Autodesk Inventor part; units mm, degrees
(part 2 of 3)
  spline S268 degree 2 poles (-6.9778, 47.9157) (-6.9778, 48.2091) (-7.3123, 48.8729) (-7.5541, 49.1508) knots 0 0 0 1 2 2 2
  line L188 (-7.5541, 49.1508) -> (-11.1151, 49.1508)
  line L189 (-11.1151, 49.1508) -> (-11.1151, 49.9535)
  line L190 (-11.1151, 49.9535) -> (-6.35, 49.9535)
  line L191 (-6.35, 54.8575) -> (-6.35, 54.0548)
  line L192 (-6.35, 54.0548) -> (-9.067, 54.0548)
  spline S269 degree 2 poles (-9.067, 54.0548) (-9.3964, 54.0548) (-9.9624, 53.993) (-10.1322, 53.9004) knots 0 0 0 1 2 2 2
  spline S270 degree 2 poles (-10.1322, 53.9004) (-10.3123, 53.8026) (-10.4873, 53.4527) (-10.4873, 53.1542) knots 0 0 0 1 2 2 2
  spline S271 degree 2 poles (-10.4873, 53.1542) (-10.4873, 52.8558) (-10.1682, 52.2228) (-9.9109, 51.9192) knots 0 0 0 1 2 2 2
  line L193 (-9.9109, 51.9192) -> (-6.35, 51.9192)
  line L194 (-6.35, 51.9192) -> (-6.35, 51.1165)
  line L195 (-6.35, 51.1165) -> (-11.1151, 51.1165)
  line L196 (-11.1151, 51.1165) -> (-11.1151, 51.9192)
  line L197 (-11.1151, 51.9192) -> (-10.585, 51.9192)
  spline S272 degree 2 poles (-10.585, 51.9192) (-10.9092, 52.2794) (-11.2489, 52.9741) (-11.2489, 53.3652) knots 0 0 0 1 2 2 2
  spline S273 degree 2 poles (-11.2489, 53.3652) (-11.2489, 54.0651) (-10.3226, 54.8575) (-9.4427, 54.8575) knots 0 0 0 1 2 2 2
  line L198 (-9.4427, 54.8575) -> (-6.35, 54.8575)
  spline S274 degree 2 poles (-6.2574, 57.4253) (-6.2574, 56.7718) (-7.0035, 56.0359) (-7.8114, 56.0359) knots 0 0 0 1 2 2 2
  line L199 (-7.8114, 56.0359) -> (-10.4513, 56.0359)
  line L200 (-10.4513, 56.0359) -> (-10.4513, 55.4956)
  line L201 (-10.4513, 55.4956) -> (-11.1151, 55.4956)
  line L202 (-11.1151, 55.4956) -> (-11.1151, 56.0359)
  line L203 (-11.1151, 56.0359) -> (-12.4839, 56.0359)
  line L204 (-12.4839, 56.0359) -> (-12.4839, 56.8387)
  line L205 (-12.4839, 56.8387) -> (-11.1151, 56.8387)
  line L206 (-11.1151, 56.8387) -> (-11.1151, 58.3155)
  line L207 (-11.1151, 58.3155) -> (-10.4513, 58.3155)
  line L208 (-10.4513, 58.3155) -> (-10.4513, 56.8387)
  line L209 (-10.4513, 56.8387) -> (-8.1819, 56.8387)
  spline S275 degree 2 poles (-8.1819, 56.8387) (-7.8217, 56.8387) (-7.4255, 56.8644) (-7.2557, 56.9519) knots 0 0 0 1 2 2 2
  spline S276 degree 2 poles (-7.2557, 56.9519) (-7.1064, 57.0239) (-6.9572, 57.3481) (-6.9572, 57.626) knots 0 0 0 1 2 2 2
  spline S277 degree 2 poles (-6.9572, 57.626) (-6.9572, 57.8215) (-7.0756, 58.1869) (-7.1116, 58.2692) knots 0 0 0 1 2 2 2
  line L210 (-7.1116, 58.2692) -> (-7.1116, 58.3155)
  line L211 (-7.1116, 58.3155) -> (-6.3912, 58.3155)
  spline S278 degree 2 poles (-6.3912, 58.3155) (-6.3294, 58.0891) (-6.2574, 57.626) (-6.2574, 57.4253) knots 0 0 0 1 2 2 2
  line L212 (-6.35, 63.5129) -> (-6.35, 62.566)
  line L213 (-6.35, 62.566) -> (-11.8252, 59.7564)
  line L214 (-11.8252, 59.7564) -> (-6.35, 59.7564)
  line L215 (-6.35, 59.7564) -> (-6.35, 58.9691)
  line L216 (-6.35, 58.9691) -> (-12.7, 58.9691)
  line L217 (-12.7, 58.9691) -> (-12.7, 60.1681)
  line L218 (-12.7, 60.1681) -> (-7.6725, 62.7255)
  line L219 (-7.6725, 62.7255) -> (-12.7, 62.7255)
  line L220 (-12.7, 62.7255) -> (-12.7, 63.5129)
  line L221 (-12.7, 63.5129) -> (-6.35, 63.5129)
  spline S279 degree 2 poles (-8.7325, 68.6536) (-7.5284, 68.6536) (-6.2162, 67.4958) (-6.2162, 66.5283) knots 0 0 0 1 2 2 2
  spline S280 degree 2 poles (-6.2162, 66.5283) (-6.2162, 65.5352) (-7.5696, 64.398) (-8.7325, 64.398) knots 0 0 0 1 2 2 2
  spline S281 degree 2 poles (-8.7325, 64.398) (-9.9264, 64.398) (-11.2489, 65.5712) (-11.2489, 66.5283) knots 0 0 0 1 2 2 2
  spline S282 degree 2 poles (-11.2489, 66.5283) (-11.2489, 67.4958) (-9.9315, 68.6536) (-8.7325, 68.6536) knots 0 0 0 1 2 2 2
  spline S283 degree 2 poles (-8.7325, 67.8251) (-9.6588, 67.8251) (-10.5593, 67.151) (-10.5593, 66.5283) knots 0 0 0 1 2 2 2
  spline S284 degree 2 poles (-10.5593, 66.5283) (-10.5593, 65.9057) (-9.6588, 65.2264) (-8.7325, 65.2264) knots 0 0 0 1 2 2 2
  spline S285 degree 2 poles (-8.7325, 65.2264) (-7.832, 65.2264) (-6.9058, 65.9057) (-6.9058, 66.5283) knots 0 0 0 1 2 2 2
  spline S286 degree 2 poles (-6.9058, 66.5283) (-6.9058, 67.1458) (-7.8166, 67.8251) (-8.7325, 67.8251) knots 0 0 0 1 2 2 2
  line L222 (-11.1151, 73.218) -> (-6.35, 71.4221)
  line L223 (-6.35, 71.4221) -> (-6.35, 70.7016)
  line L224 (-6.35, 70.7016) -> (-11.1151, 68.9212)
  line L225 (-11.1151, 68.9212) -> (-11.1151, 69.7908)
  line L226 (-11.1151, 69.7908) -> (-7.4461, 71.0927)
  line L227 (-7.4461, 71.0927) -> (-11.1151, 72.3843)
  line L228 (-11.1151, 72.3843) -> (-11.1151, 73.218)
  line L229 (-6.35, 77.6228) -> (-6.35, 73.7068)
  line L230 (-6.35, 73.7068) -> (-7.2505, 73.7068)
  spline S287 degree 2 poles (-7.2505, 73.7068) (-7.6468, 74.1288) (-8.3826, 74.8801) (-8.7788, 75.2403) knots 0 0 0 1 2 2 2
  spline S288 degree 2 poles (-8.7788, 75.2403) (-9.5765, 75.9659) (-10.5336, 76.4959) (-11.043, 76.4959) knots 0 0 0 1 2 2 2
  spline S289 degree 2 poles (-11.043, 76.4959) (-11.3106, 76.4959) (-11.712, 76.3312) (-11.8406, 76.182) knots 0 0 0 1 2 2 2
  spline S290 degree 2 poles (-11.8406, 76.182) (-11.9693, 76.0328) (-12.0979, 75.6417) (-12.0979, 75.405) knots 0 0 0 1 2 2 2
  spline S291 degree 2 poles (-12.0979, 75.405) (-12.0979, 75.1785) (-11.9847, 74.7154) (-11.8972, 74.5044) knots 0 0 0 1 2 2 2
  spline S292 degree 2 poles (-11.8972, 74.5044) (-11.8252, 74.3243) (-11.6194, 73.9899) (-11.5473, 73.8869) knots 0 0 0 1 2 2 2
  line L231 (-11.5473, 73.8869) -> (-11.5473, 73.8406)
  line L232 (-11.5473, 73.8406) -> (-12.453, 73.8406)
  spline S293 degree 2 poles (-12.453, 73.8406) (-12.5816, 74.1031) (-12.8338, 75.0448) (-12.8338, 75.4667) knots 0 0 0 1 2 2 2
  spline S294 degree 2 poles (-12.8338, 75.4667) (-12.8338, 76.3569) (-11.8921, 77.3604) (-11.0893, 77.3604) knots 0 0 0 1 2 2 2
  spline S295 degree 2 poles (-11.0893, 77.3604) (-10.7137, 77.3604) (-10.0859, 77.1854) (-9.8183, 77.0311) knots 0 0 0 1 2 2 2
  spline S296 degree 2 poles (-9.8183, 77.0311) (-9.5404, 76.8767) (-8.995, 76.429) (-8.7325, 76.182) knots 0 0 0 1 2 2 2
  spline S297 degree 2 poles (-8.7325, 76.182) (-8.2951, 75.7806) (-7.3586, 74.7978) (-7.0859, 74.5044) knots 0 0 0 1 2 2 2
  line L233 (-7.0859, 74.5044) -> (-7.0859, 77.6228)
  line L234 (-7.0859, 77.6228) -> (-6.35, 77.6228)
  spline S298 degree 2 poles (-9.525, 82.4239) (-7.8166, 82.4239) (-6.2162, 81.4308) (-6.2162, 80.3965) knots 0 0 0 1 2 2 2
  spline S299 degree 2 poles (-6.2162, 80.3965) (-6.2162, 79.3467) (-7.8474, 78.3638) (-9.5199, 78.3638) knots 0 0 0 1 2 2 2
  spline S300 degree 2 poles (-9.5199, 78.3638) (-11.2386, 78.3638) (-12.8286, 79.357) (-12.8286, 80.3965) knots 0 0 0 1 2 2 2
  spline S301 degree 2 poles (-12.8286, 80.3965) (-12.8286, 81.4411) (-11.182, 82.4239) (-9.525, 82.4239) knots 0 0 0 1 2 2 2
  spline S302 degree 2 poles (-7.5902, 81.333) (-7.9041, 81.4565) (-8.8715, 81.5594) (-9.525, 81.5594) knots 0 0 0 1 2 2 2
  spline S303 degree 2 poles (-9.525, 81.5594) (-10.1785, 81.5594) (-11.1408, 81.4565) (-11.465, 81.3279) knots 0 0 0 1 2 2 2
  spline S304 degree 2 poles (-11.465, 81.3279) (-11.7892, 81.1992) (-12.1237, 80.7515) (-12.1237, 80.3965) knots 0 0 0 1 2 2 2
  spline S305 degree 2 poles (-12.1237, 80.3965) (-12.1237, 80.0414) (-11.7892, 79.5834) (-11.4547, 79.4496) knots 0 0 0 1 2 2 2
  spline S306 degree 2 poles (-11.4547, 79.4496) (-11.1305, 79.321) (-10.1425, 79.2283) (-9.5199, 79.2283) knots 0 0 0 1 2 2 2
  spline S307 degree 2 poles (-9.5199, 79.2283) (-8.8509, 79.2283) (-7.9555, 79.3107) (-7.6056, 79.4445) knots 0 0 0 1 2 2 2
  spline S308 degree 2 poles (-7.6056, 79.4445) (-7.2763, 79.568) (-6.9212, 80.026) (-6.9212, 80.3965) knots 0 0 0 1 2 2 2
  spline S309 degree 2 poles (-6.9212, 80.3965) (-6.9212, 80.7464) (-7.2557, 81.2044) (-7.5902, 81.333) knots 0 0 0 1 2 2 2
  line L235 (-6.35, 87.153) -> (-6.35, 83.237)
  line L236 (-6.35, 83.237) -> (-7.2505, 83.237)
  spline S310 degree 2 poles (-7.2505, 83.237) (-7.6468, 83.6589) (-8.3826, 84.4102) (-8.7788, 84.7704) knots 0 0 0 1 2 2 2
  spline S311 degree 2 poles (-8.7788, 84.7704) (-9.5765, 85.496) (-10.5336, 86.026) (-11.043, 86.026) knots 0 0 0 1 2 2 2
  spline S312 degree 2 poles (-11.043, 86.026) (-11.3106, 86.026) (-11.712, 85.8614) (-11.8406, 85.7121) knots 0 0 0 1 2 2 2
  spline S313 degree 2 poles (-11.8406, 85.7121) (-11.9693, 85.5629) (-12.0979, 85.1718) (-12.0979, 84.9351) knots 0 0 0 1 2 2 2
  spline S314 degree 2 poles (-12.0979, 84.9351) (-12.0979, 84.7087) (-11.9847, 84.2456) (-11.8972, 84.0346) knots 0 0 0 1 2 2 2
  spline S315 degree 2 poles (-11.8972, 84.0346) (-11.8252, 83.8545) (-11.6194, 83.52) (-11.5473, 83.4171) knots 0 0 0 1 2 2 2
  line L237 (-11.5473, 83.4171) -> (-11.5473, 83.3708)
  line L238 (-11.5473, 83.3708) -> (-12.453, 83.3708)
  spline S316 degree 2 poles (-12.453, 83.3708) (-12.5816, 83.6332) (-12.8338, 84.5749) (-12.8338, 84.9969) knots 0 0 0 1 2 2 2
  spline S317 degree 2 poles (-12.8338, 84.9969) (-12.8338, 85.8871) (-11.8921, 86.8905) (-11.0893, 86.8905) knots 0 0 0 1 2 2 2
  spline S318 degree 2 poles (-11.0893, 86.8905) (-10.7137, 86.8905) (-10.0859, 86.7156) (-9.8183, 86.5612) knots 0 0 0 1 2 2 2
  spline S319 degree 2 poles (-9.8183, 86.5612) (-9.5404, 86.4068) (-8.995, 85.9591) (-8.7325, 85.7121) knots 0 0 0 1 2 2 2
  spline S320 degree 2 poles (-8.7325, 85.7121) (-8.2951, 85.3108) (-7.3586, 84.3279) (-7.0859, 84.0346) knots 0 0 0 1 2 2 2
  line L239 (-7.0859, 84.0346) -> (-7.0859, 87.153)
  line L240 (-7.0859, 87.153) -> (-6.35, 87.153)
  spline S321 degree 2 poles (-9.525, 91.9541) (-7.8166, 91.9541) (-6.2162, 90.9609) (-6.2162, 89.9266) knots 0 0 0 1 2 2 2
  spline S322 degree 2 poles (-6.2162, 89.9266) (-6.2162, 88.8768) (-7.8474, 87.894) (-9.5199, 87.894) knots 0 0 0 1 2 2 2
  spline S323 degree 2 poles (-9.5199, 87.894) (-11.2386, 87.894) (-12.8286, 88.8871) (-12.8286, 89.9266) knots 0 0 0 1 2 2 2
  spline S324 degree 2 poles (-12.8286, 89.9266) (-12.8286, 90.9712) (-11.182, 91.9541) (-9.525, 91.9541) knots 0 0 0 1 2 2 2
  spline S325 degree 2 poles (-7.5902, 90.8631) (-7.9041, 90.9866) (-8.8715, 91.0896) (-9.525, 91.0896) knots 0 0 0 1 2 2 2
  spline S326 degree 2 poles (-9.525, 91.0896) (-10.1785, 91.0896) (-11.1408, 90.9866) (-11.465, 90.858) knots 0 0 0 1 2 2 2
  spline S327 degree 2 poles (-11.465, 90.858) (-11.7892, 90.7294) (-12.1237, 90.2817) (-12.1237, 89.9266) knots 0 0 0 1 2 2 2
  spline S328 degree 2 poles (-12.1237, 89.9266) (-12.1237, 89.5715) (-11.7892, 89.1136) (-11.4547, 88.9798) knots 0 0 0 1 2 2 2
  spline S329 degree 2 poles (-11.4547, 88.9798) (-11.1305, 88.8511) (-10.1425, 88.7585) (-9.5199, 88.7585) knots 0 0 0 1 2 2 2
  spline S330 degree 2 poles (-9.5199, 88.7585) (-8.8509, 88.7585) (-7.9555, 88.8408) (-7.6056, 88.9746) knots 0 0 0 1 2 2 2
  spline S331 degree 2 poles (-7.6056, 88.9746) (-7.2763, 89.0981) (-6.9212, 89.5561) (-6.9212, 89.9266) knots 0 0 0 1 2 2 2
  spline S332 degree 2 poles (-6.9212, 89.9266) (-6.9212, 90.2765) (-7.2557, 90.7345) (-7.5902, 90.8631) knots 0 0 0 1 2 2 2
  line L241 (-1.5346, -65.6741) -> (-1.5346, -65.7153)
  spline S333 degree 2 poles (-1.5346, -65.7153) (-1.5758, -65.8234) (-1.6478, -66.2247) (-1.6478, -66.3843) knots 0 0 0 1 2 2 2
  spline S334 degree 2 poles (-1.6478, -66.3843) (-1.6478, -66.8885) (-1.195, -67.3208) (-0.5981, -67.3208) knots 0 0 0 1 2 2 2
  line L242 (-0.5981, -67.3208) -> (-0.4385, -67.3208)
  line L243 (-0.4385, -67.3208) -> (-0.4385, -65.9932)
  line L244 (-0.4385, -65.9932) -> (0.2253, -65.9932)
  line L245 (0.2253, -65.9932) -> (0.2253, -67.2951)
  line L246 (0.2253, -67.2951) -> (4.3265, -67.2951)
  line L247 (4.3265, -67.2951) -> (4.3265, -68.0978)
  line L248 (4.3265, -68.0978) -> (0.2253, -68.0978)
  line L249 (0.2253, -68.0978) -> (0.2253, -68.6381)
  line L250 (0.2253, -68.6381) -> (-0.4385, -68.6381)
  line L251 (-0.4385, -68.6381) -> (-0.4385, -68.0978)
  line L252 (-0.4385, -68.0978) -> (-0.5981, -68.0978)
  spline S335 degree 2 poles (-0.5981, -68.0978) (-1.4523, -68.0978) (-2.3477, -67.2693) (-2.3477, -66.4975) knots 0 0 0 1 2 2 2
  spline S336 degree 2 poles (-2.3477, -66.4975) (-2.3477, -66.2762) (-2.3013, -65.8491) (-2.2705, -65.6741) knots 0 0 0 1 2 2 2
  line L253 (-2.2705, -65.6741) -> (-1.5346, -65.6741)
  line L254 (4.3265, -64.3979) -> (4.3265, -65.2007)
  line L255 (4.3265, -65.2007) -> (-0.4385, -65.2007)
  line L256 (-0.4385, -65.2007) -> (-0.4385, -64.3979)
  line L257 (-0.4385, -64.3979) -> (4.3265, -64.3979)
  line L258 (-1.231, -64.3413) -> (-1.231, -65.2522)
  line L259 (-1.231, -65.2522) -> (-2.0646, -65.2522)
  line L260 (-2.0646, -65.2522) -> (-2.0646, -64.3413)
  line L261 (-2.0646, -64.3413) -> (-1.231, -64.3413)
  line L262 (4.3265, -62.4014) -> (4.3265, -63.2041)
  line L263 (4.3265, -63.2041) -> (-2.3065, -63.2041)
  line L264 (-2.3065, -63.2041) -> (-2.3065, -62.4014)
  line L265 (-2.3065, -62.4014) -> (4.3265, -62.4014)
  spline S337 degree 2 poles (4.4346, -59.1543) (4.4346, -60.2967) (3.1533, -61.5523) (1.9697, -61.5523) knots 0 0 0 1 2 2 2
  spline S338 degree 2 poles (1.9697, -61.5523) (0.8068, -61.5523) (-0.5723, -60.3327) (-0.5723, -59.3499) knots 0 0 0 1 2 2 2
  spline S339 degree 2 poles (-0.5723, -59.3499) (-0.5723, -58.9073) (-0.315, -58.2229) (-0.0423, -57.9708) knots 0 0 0 1 2 2 2
  spline S340 degree 2 poles (-0.0423, -57.9708) (0.2304, -57.7135) (1.0177, -57.4407) (1.5889, -57.4407) knots 0 0 0 1 2 2 2
  line L266 (1.5889, -57.4407) -> (2.0263, -57.4407)
  line L267 (2.0263, -57.4407) -> (2.0263, -60.7392)
  spline S341 degree 2 poles (2.0263, -60.7392) (2.8548, -60.7392) (3.7348, -59.9056) (3.7348, -59.1646) knots 0 0 0 1 2 2 2
  spline S342 degree 2 poles (3.7348, -59.1646) (3.7348, -58.9022) (3.6164, -58.3927) (3.5238, -58.1869) knots 0 0 0 1 2 2 2
  spline S343 degree 2 poles (3.5238, -58.1869) (3.4209, -57.9708) (3.2408, -57.6723) (3.1584, -57.5745) knots 0 0 0 1 2 2 2
  line L268 (3.1584, -57.5745) -> (3.1584, -57.5282)
  line L269 (3.1584, -57.5282) -> (4.0332, -57.5282)
  spline S344 degree 2 poles (4.0332, -57.5282) (4.0898, -57.6672) (4.2545, -58.0891) (4.3008, -58.2538) knots 0 0 0 1 2 2 2
  spline S345 degree 2 poles (4.3008, -58.2538) (4.3677, -58.4853) (4.4346, -58.8661) (4.4346, -59.1543) knots 0 0 0 1 2 2 2
  spline S346 degree 2 poles (1.414, -58.2229) (1.0898, -58.2332) (0.6164, -58.367) (0.4568, -58.4956) knots 0 0 0 1 2 2 2
  spline S347 degree 2 poles (0.4568, -58.4956) (0.2767, -58.6346) (0.0863, -59.072) (0.0863, -59.3962) knots 0 0 0 1 2 2 2
  spline S348 degree 2 poles (0.0863, -59.3962) (0.0863, -59.7152) (0.2767, -60.1629) (0.462, -60.3482) knots 0 0 0 1 2 2 2
  spline S349 degree 2 poles (0.462, -60.3482) (0.6524, -60.5283) (1.1104, -60.7135) (1.414, -60.7392) knots 0 0 0 1 2 2 2
  line L270 (1.414, -60.7392) -> (1.414, -58.2229)
  line L271 (4.3265, -55.156) -> (4.3265, -56.1749)
  line L272 (4.3265, -56.1749) -> (3.1121, -56.1749)
  line L273 (3.1121, -56.1749) -> (3.1121, -55.156)
  line L274 (3.1121, -55.156) -> (4.3265, -55.156)
  line L275 (0.7759, -55.156) -> (0.7759, -56.1749)
  line L276 (0.7759, -56.1749) -> (-0.4385, -56.1749)
  line L277 (-0.4385, -56.1749) -> (-0.4385, -55.156)
  line L278 (-0.4385, -55.156) -> (0.7759, -55.156)
  spline S350 degree 2 poles (4.4346, -48.9192) (4.4346, -49.4132) (4.131, -50.2314) (3.8222, -50.5247) knots 0 0 0 1 2 2 2
  spline S351 degree 2 poles (3.8222, -50.5247) (3.5186, -50.818) (2.5821, -51.1422) (1.9543, -51.1422) knots 0 0 0 1 2 2 2
  spline S352 degree 2 poles (1.9543, -51.1422) (1.3265, -51.1422) (0.4105, -50.8077) (0.1018, -50.5247) knots 0 0 0 1 2 2 2
  spline S353 degree 2 poles (0.1018, -50.5247) (-0.2121, -50.2417) (-0.5466, -49.4029) (-0.5466, -48.9192) knots 0 0 0 1 2 2 2
  spline S354 degree 2 poles (-0.5466, -48.9192) (-0.5466, -48.5281) (-0.3253, -47.7974) (-0.1813, -47.5144) knots 0 0 0 1 2 2 2
  line L279 (-0.1813, -47.5144) -> (0.7193, -47.5144)
  line L280 (0.7193, -47.5144) -> (0.7193, -47.5607)
  spline S355 degree 2 poles (0.7193, -47.5607) (0.6472, -47.6482) (0.462, -47.9157) (0.3642, -48.1061) knots 0 0 0 1 2 2 2
  spline S356 degree 2 poles (0.3642, -48.1061) (0.2819, -48.2759) (0.1532, -48.7288) (0.1532, -48.9346) knots 0 0 0 1 2 2 2
  spline S357 degree 2 poles (0.1532, -48.9346) (0.1532, -49.5573) (1.0949, -50.3137) (1.9543, -50.3137) knots 0 0 0 1 2 2 2
  spline S358 degree 2 poles (1.9543, -50.3137) (2.7931, -50.3137) (3.7348, -49.583) (3.7348, -48.9346) knots 0 0 0 1 2 2 2
  spline S359 degree 2 poles (3.7348, -48.9346) (3.7348, -48.5435) (3.4106, -47.8334) (3.1584, -47.5607) knots 0 0 0 1 2 2 2
  line L281 (3.1584, -47.5607) -> (3.1584, -47.5144)
  line L282 (3.1584, -47.5144) -> (4.0589, -47.5144)
  spline S360 degree 2 poles (4.0589, -47.5144) (4.1155, -47.6327) (4.2751, -47.9929) (4.3111, -48.137) knots 0 0 0 1 2 2 2
  spline S361 degree 2 poles (4.3111, -48.137) (4.3728, -48.3428) (4.4346, -48.667) (4.4346, -48.9192) knots 0 0 0 1 2 2 2
  spline S362 degree 2 poles (1.944, -42.8676) (3.1481, -42.8676) (4.4603, -44.0255) (4.4603, -44.9929) knots 0 0 0 1 2 2 2
  spline S363 degree 2 poles (4.4603, -44.9929) (4.4603, -45.986) (3.107, -47.1233) (1.944, -47.1233) knots 0 0 0 1 2 2 2
  spline S364 degree 2 poles (1.944, -47.1233) (0.7502, -47.1233) (-0.5723, -45.95) (-0.5723, -44.9929) knots 0 0 0 1 2 2 2
  spline S365 degree 2 poles (-0.5723, -44.9929) (-0.5723, -44.0255) (0.745, -42.8676) (1.944, -42.8676) knots 0 0 0 1 2 2 2
  spline S366 degree 2 poles (1.944, -43.6961) (1.0177, -43.6961) (0.1172, -44.3702) (0.1172, -44.9929) knots 0 0 0 1 2 2 2
  spline S367 degree 2 poles (0.1172, -44.9929) (0.1172, -45.6155) (1.0177, -46.2948) (1.944, -46.2948) knots 0 0 0 1 2 2 2
  spline S368 degree 2 poles (1.944, -46.2948) (2.8445, -46.2948) (3.7708, -45.6155) (3.7708, -44.9929) knots 0 0 0 1 2 2 2
  spline S369 degree 2 poles (3.7708, -44.9929) (3.7708, -44.3754) (2.86, -43.6961) (1.944, -43.6961) knots 0 0 0 1 2 2 2
  line L283 (4.3265, -38.3033) -> (4.3265, -39.106)
  line L284 (4.3265, -39.106) -> (1.6095, -39.106)
  spline S370 degree 2 poles (1.6095, -39.106) (1.2802, -39.106) (0.7141, -39.1678) (0.5443, -39.2604) knots 0 0 0 1 2 2 2
  spline S371 degree 2 poles (0.5443, -39.2604) (0.3642, -39.3582) (0.1893, -39.7081) (0.1893, -40.0065) knots 0 0 0 1 2 2 2
  spline S372 degree 2 poles (0.1893, -40.0065) (0.1893, -40.305) (0.5083, -40.9379) (0.7656, -41.2415) knots 0 0 0 1 2 2 2
  line L285 (0.7656, -41.2415) -> (4.3265, -41.2415)
  line L286 (4.3265, -41.2415) -> (4.3265, -42.0443)
  line L287 (4.3265, -42.0443) -> (-0.4385, -42.0443)
  line L288 (-0.4385, -42.0443) -> (-0.4385, -41.2415)
  line L289 (-0.4385, -41.2415) -> (0.0915, -41.2415)
  spline S373 degree 2 poles (0.0915, -41.2415) (-0.2327, -40.8813) (-0.5723, -40.1866) (-0.5723, -39.7956) knots 0 0 0 1 2 2 2
  spline S374 degree 2 poles (-0.5723, -39.7956) (-0.5723, -39.0957) (0.3539, -38.3033) (1.2339, -38.3033) knots 0 0 0 1 2 2 2
  line L290 (1.2339, -38.3033) -> (4.3265, -38.3033)
  line L291 (4.3265, -33.4353) -> (4.3265, -34.238)
  line L292 (4.3265, -34.238) -> (1.6095, -34.238)
  spline S375 degree 2 poles (1.6095, -34.238) (1.2802, -34.238) (0.7141, -34.2998) (0.5443, -34.3924) knots 0 0 0 1 2 2 2
  spline S376 degree 2 poles (0.5443, -34.3924) (0.3642, -34.4902) (0.1893, -34.8401) (0.1893, -35.1386) knots 0 0 0 1 2 2 2
  spline S377 degree 2 poles (0.1893, -35.1386) (0.1893, -35.437) (0.5083, -36.07) (0.7656, -36.3736) knots 0 0 0 1 2 2 2
  line L293 (0.7656, -36.3736) -> (4.3265, -36.3736)
  line L294 (4.3265, -36.3736) -> (4.3265, -37.1763)
  line L295 (4.3265, -37.1763) -> (-0.4385, -37.1763)
  line L296 (-0.4385, -37.1763) -> (-0.4385, -36.3736)
  line L297 (-0.4385, -36.3736) -> (0.0915, -36.3736)
  spline S378 degree 2 poles (0.0915, -36.3736) (-0.2327, -36.0133) (-0.5723, -35.3187) (-0.5723, -34.9276) knots 0 0 0 1 2 2 2
  spline S379 degree 2 poles (-0.5723, -34.9276) (-0.5723, -34.2277) (0.3539, -33.4353) (1.2339, -33.4353) knots 0 0 0 1 2 2 2
  line L298 (1.2339, -33.4353) -> (4.3265, -33.4353)
  spline S380 degree 2 poles (4.4346, -30.2397) (4.4346, -31.3821) (3.1533, -32.6377) (1.9697, -32.6377) knots 0 0 0 1 2 2 2
  spline S381 degree 2 poles (1.9697, -32.6377) (0.8068, -32.6377) (-0.5723, -31.4181) (-0.5723, -30.4352) knots 0 0 0 1 2 2 2
  spline S382 degree 2 poles (-0.5723, -30.4352) (-0.5723, -29.9927) (-0.315, -29.3083) (-0.0423, -29.0561) knots 0 0 0 1 2 2 2
  spline S383 degree 2 poles (-0.0423, -29.0561) (0.2304, -28.7988) (1.0177, -28.5261) (1.5889, -28.5261) knots 0 0 0 1 2 2 2
  line L299 (1.5889, -28.5261) -> (2.0263, -28.5261)
  line L300 (2.0263, -28.5261) -> (2.0263, -31.8246)
  spline S384 degree 2 poles (2.0263, -31.8246) (2.8548, -31.8246) (3.7348, -30.991) (3.7348, -30.25) knots 0 0 0 1 2 2 2
  spline S385 degree 2 poles (3.7348, -30.25) (3.7348, -29.9875) (3.6164, -29.4781) (3.5238, -29.2723) knots 0 0 0 1 2 2 2
  spline S386 degree 2 poles (3.5238, -29.2723) (3.4209, -29.0561) (3.2408, -28.7577) (3.1584, -28.6599) knots 0 0 0 1 2 2 2
  line L301 (3.1584, -28.6599) -> (3.1584, -28.6136)
  line L302 (3.1584, -28.6136) -> (4.0332, -28.6136)
  spline S387 degree 2 poles (4.0332, -28.6136) (4.0898, -28.7525) (4.2545, -29.1745) (4.3008, -29.3392) knots 0 0 0 1 2 2 2
  spline S388 degree 2 poles (4.3008, -29.3392) (4.3677, -29.5707) (4.4346, -29.9515) (4.4346, -30.2397) knots 0 0 0 1 2 2 2
  spline S389 degree 2 poles (1.414, -29.3083) (1.0898, -29.3186) (0.6164, -29.4524) (0.4568, -29.581) knots 0 0 0 1 2 2 2
  spline S390 degree 2 poles (0.4568, -29.581) (0.2767, -29.72) (0.0863, -30.1574) (0.0863, -30.4815) knots 0 0 0 1 2 2 2
  spline S391 degree 2 poles (0.0863, -30.4815) (0.0863, -30.8006) (0.2767, -31.2483) (0.462, -31.4335) knots 0 0 0 1 2 2 2
  spline S392 degree 2 poles (0.462, -31.4335) (0.6524, -31.6136) (1.1104, -31.7989) (1.414, -31.8246) knots 0 0 0 1 2 2 2
  line L303 (1.414, -31.8246) -> (1.414, -29.3083)
  spline S393 degree 2 poles (4.4346, -25.8194) (4.4346, -26.3134) (4.131, -27.1316) (3.8222, -27.4249) knots 0 0 0 1 2 2 2
  spline S394 degree 2 poles (3.8222, -27.4249) (3.5186, -27.7182) (2.5821, -28.0424) (1.9543, -28.0424) knots 0 0 0 1 2 2 2
  spline S395 degree 2 poles (1.9543, -28.0424) (1.3265, -28.0424) (0.4105, -27.7079) (0.1018, -27.4249) knots 0 0 0 1 2 2 2
  spline S396 degree 2 poles (0.1018, -27.4249) (-0.2121, -27.1419) (-0.5466, -26.3031) (-0.5466, -25.8194) knots 0 0 0 1 2 2 2
  spline S397 degree 2 poles (-0.5466, -25.8194) (-0.5466, -25.4283) (-0.3253, -24.6976) (-0.1813, -24.4146) knots 0 0 0 1 2 2 2
  line L304 (-0.1813, -24.4146) -> (0.7193, -24.4146)
  line L305 (0.7193, -24.4146) -> (0.7193, -24.4609)
  spline S398 degree 2 poles (0.7193, -24.4609) (0.6472, -24.5484) (0.462, -24.8159) (0.3642, -25.0063) knots 0 0 0 1 2 2 2
  spline S399 degree 2 poles (0.3642, -25.0063) (0.2819, -25.1762) (0.1532, -25.629) (0.1532, -25.8348) knots 0 0 0 1 2 2 2
  spline S400 degree 2 poles (0.1532, -25.8348) (0.1532, -26.4575) (1.0949, -27.2139) (1.9543, -27.2139) knots 0 0 0 1 2 2 2
  spline S401 degree 2 poles (1.9543, -27.2139) (2.7931, -27.2139) (3.7348, -26.4832) (3.7348, -25.8348) knots 0 0 0 1 2 2 2
  spline S402 degree 2 poles (3.7348, -25.8348) (3.7348, -25.4437) (3.4106, -24.7336) (3.1584, -24.4609) knots 0 0 0 1 2 2 2
  line L306 (3.1584, -24.4609) -> (3.1584, -24.4146)
  line L307 (3.1584, -24.4146) -> (4.0589, -24.4146)
  spline S403 degree 2 poles (4.0589, -24.4146) (4.1155, -24.5329) (4.2751, -24.8931) (4.3111, -25.0372) knots 0 0 0 1 2 2 2
  spline S404 degree 2 poles (4.3111, -25.0372) (4.3728, -25.243) (4.4346, -25.5672) (4.4346, -25.8194) knots 0 0 0 1 2 2 2
  spline S405 degree 2 poles (4.4192, -22.243) (4.4192, -22.8965) (3.673, -23.6324) (2.8651, -23.6324) knots 0 0 0 1 2 2 2
  line L308 (2.8651, -23.6324) -> (0.2253, -23.6324)
  line L309 (0.2253, -23.6324) -> (0.2253, -24.1727)
  line L310 (0.2253, -24.1727) -> (-0.4385, -24.1727)
  line L311 (-0.4385, -24.1727) -> (-0.4385, -23.6324)
  line L312 (-0.4385, -23.6324) -> (-1.8073, -23.6324)
  line L313 (-1.8073, -23.6324) -> (-1.8073, -22.8296)
  line L314 (-1.8073, -22.8296) -> (-0.4385, -22.8296)
  line L315 (-0.4385, -22.8296) -> (-0.4385, -21.3528)
  line L316 (-0.4385, -21.3528) -> (0.2253, -21.3528)
  line L317 (0.2253, -21.3528) -> (0.2253, -22.8296)
  line L318 (0.2253, -22.8296) -> (2.4946, -22.8296)
  spline S406 degree 2 poles (2.4946, -22.8296) (2.8548, -22.8296) (3.251, -22.8039) (3.4209, -22.7164) knots 0 0 0 1 2 2 2
  spline S407 degree 2 poles (3.4209, -22.7164) (3.5701, -22.6444) (3.7193, -22.3202) (3.7193, -22.0423) knots 0 0 0 1 2 2 2
  spline S408 degree 2 poles (3.7193, -22.0423) (3.7193, -21.8468) (3.601, -21.4814) (3.5649, -21.3991) knots 0 0 0 1 2 2 2
  line L319 (3.5649, -21.3991) -> (3.5649, -21.3528)
  line L320 (3.5649, -21.3528) -> (4.2854, -21.3528)
  spline S409 degree 2 poles (4.2854, -21.3528) (4.3471, -21.5792) (4.4192, -22.0423) (4.4192, -22.243) knots 0 0 0 1 2 2 2
  spline S410 degree 2 poles (1.944, -16.845) (3.1481, -16.845) (4.4603, -18.0028) (4.4603, -18.9702) knots 0 0 0 1 2 2 2
  spline S411 degree 2 poles (4.4603, -18.9702) (4.4603, -19.9634) (3.107, -21.1006) (1.944, -21.1006) knots 0 0 0 1 2 2 2
  spline S412 degree 2 poles (1.944, -21.1006) (0.7502, -21.1006) (-0.5723, -19.9274) (-0.5723, -18.9702) knots 0 0 0 1 2 2 2
  spline S413 degree 2 poles (-0.5723, -18.9702) (-0.5723, -18.0028) (0.745, -16.845) (1.944, -16.845) knots 0 0 0 1 2 2 2
  spline S414 degree 2 poles (1.944, -17.6735) (1.0177, -17.6735) (0.1172, -18.3476) (0.1172, -18.9702) knots 0 0 0 1 2 2 2
  spline S415 degree 2 poles (0.1172, -18.9702) (0.1172, -19.5929) (1.0177, -20.2721) (1.944, -20.2721) knots 0 0 0 1 2 2 2
  spline S416 degree 2 poles (1.944, -20.2721) (2.8445, -20.2721) (3.7708, -19.5929) (3.7708, -18.9702) knots 0 0 0 1 2 2 2
  spline S417 degree 2 poles (3.7708, -18.9702) (3.7708, -18.3527) (2.86, -17.6735) (1.944, -17.6735) knots 0 0 0 1 2 2 2
  line L321 (0.4208, -13.495) -> (0.4208, -13.5362)
  spline S418 degree 2 poles (0.4208, -13.5362) (0.3951, -13.6288) (0.3848, -13.8295) (0.3848, -13.9685) knots 0 0 0 1 2 2 2
  spline S419 degree 2 poles (0.3848, -13.9685) (0.3848, -14.2926) (0.6678, -14.9307) (0.9457, -15.2189) knots 0 0 0 1 2 2 2
  line L322 (0.9457, -15.2189) -> (4.3265, -15.2189)
  line L323 (4.3265, -15.2189) -> (4.3265, -16.0217)
  line L324 (4.3265, -16.0217) -> (-0.4385, -16.0217)
  line L325 (-0.4385, -16.0217) -> (-0.4385, -15.2189)
  line L326 (-0.4385, -15.2189) -> (0.2716, -15.2189)
  spline S420 degree 2 poles (0.2716, -15.2189) (-0.1195, -14.7815) (-0.4385, -14.128) (-0.4385, -13.8192) knots 0 0 0 1 2 2 2
  spline S421 degree 2 poles (-0.4385, -13.8192) (-0.4385, -13.6957) (-0.4283, -13.5722) (-0.4128, -13.495) knots 0 0 0 1 2 2 2
  line L327 (-0.4128, -13.495) -> (0.4208, -13.495)
  line L328 (4.3265, -11.3286) -> (-1.2722, -11.3286)
  line L329 (-1.2722, -11.3286) -> (-1.2722, -13.459)
  line L330 (-1.2722, -13.459) -> (-2.0235, -13.459)
  line L331 (-2.0235, -13.459) -> (-2.0235, -8.3543)
  line L332 (-2.0235, -8.3543) -> (-1.2722, -8.3543)
  line L333 (-1.2722, -8.3543) -> (-1.2722, -10.4847)
  line L334 (-1.2722, -10.4847) -> (4.3265, -10.4847)
  line L335 (4.3265, -10.4847) -> (4.3265, -11.3286)
  spline S422 degree 2 poles (1.944, -3.8517) (3.1481, -3.8517) (4.4603, -5.0095) (4.4603, -5.9769) knots 0 0 0 1 2 2 2
  spline S423 degree 2 poles (4.4603, -5.9769) (4.4603, -6.9701) (3.107, -8.1073) (1.944, -8.1073) knots 0 0 0 1 2 2 2
  spline S424 degree 2 poles (1.944, -8.1073) (0.7502, -8.1073) (-0.5723, -6.9341) (-0.5723, -5.9769) knots 0 0 0 1 2 2 2
  spline S425 degree 2 poles (-0.5723, -5.9769) (-0.5723, -5.0095) (0.745, -3.8517) (1.944, -3.8517) knots 0 0 0 1 2 2 2
  spline S426 degree 2 poles (1.944, -4.6802) (1.0177, -4.6802) (0.1172, -5.3543) (0.1172, -5.9769) knots 0 0 0 1 2 2 2
  spline S427 degree 2 poles (0.1172, -5.9769) (0.1172, -6.5996) (1.0177, -7.2788) (1.944, -7.2788) knots 0 0 0 1 2 2 2
  spline S428 degree 2 poles (1.944, -7.2788) (2.8445, -7.2788) (3.7708, -6.5996) (3.7708, -5.9769) knots 0 0 0 1 2 2 2
  spline S429 degree 2 poles (3.7708, -5.9769) (3.7708, -5.3594) (2.86, -4.6802) (1.944, -4.6802) knots 0 0 0 1 2 2 2
  line L336 (4.3265, -1.4846) -> (-1.2722, -1.4846)
  line L337 (-1.2722, -1.4846) -> (-1.2722, -3.615)
  line L338 (-1.2722, -3.615) -> (-2.0235, -3.615)
  line L339 (-2.0235, -3.615) -> (-2.0235, 1.4897)
  line L340 (-2.0235, 1.4897) -> (-1.2722, 1.4897)
  line L341 (-1.2722, 1.4897) -> (-1.2722, -0.6407)
  line L342 (-1.2722, -0.6407) -> (4.3265, -0.6407)
  line L343 (4.3265, -0.6407) -> (4.3265, -1.4846)
  line L344 (4.3265, 5.7814) -> (4.3265, 4.9786)
  line L345 (4.3265, 4.9786) -> (3.8016, 4.9786)
  spline S430 degree 2 poles (3.8016, 4.9786) (4.1258, 4.6081) (4.4603, 3.9443) (4.4603, 3.5326) knots 0 0 0 1 2 2 2
  spline S431 degree 2 poles (4.4603, 3.5326) (4.4603, 3.2239) (4.2545, 2.6733) (4.0332, 2.4726) knots 0 0 0 1 2 2 2
  spline S432 degree 2 poles (4.0332, 2.4726) (3.8119, 2.2668) (3.1378, 2.0403) (2.6541, 2.0403) knots 0 0 0 1 2 2 2
  line L346 (2.6541, 2.0403) -> (-0.4385, 2.0403)
  line L347 (-0.4385, 2.0403) -> (-0.4385, 2.8431)
  line L348 (-0.4385, 2.8431) -> (2.2785, 2.8431)
  spline S433 degree 2 poles (2.2785, 2.8431) (2.6593, 2.8431) (3.1584, 2.8997) (3.3437, 2.9975) knots 0 0 0 1 2 2 2
  spline S434 degree 2 poles (3.3437, 2.9975) (3.5289, 3.0952) (3.6987, 3.4297) (3.6987, 3.7436) knots 0 0 0 1 2 2 2
  spline S435 degree 2 poles (3.6987, 3.7436) (3.6987, 4.0369) (3.3643, 4.7008) (3.1224, 4.9786) knots 0 0 0 1 2 2 2
  line L349 (3.1224, 4.9786) -> (-0.4385, 4.9786)
  line L350 (-0.4385, 4.9786) -> (-0.4385, 5.7814)
  line L351 (-0.4385, 5.7814) -> (4.3265, 5.7814)
  spline S436 degree 2 poles (1.8668, 10.9375) (3.0349, 10.9375) (4.4603, 9.8055) (4.4603, 8.9512) knots 0 0 0 1 2 2 2
  spline S437 degree 2 poles (4.4603, 8.9512) (4.4603, 8.5653) (4.2699, 8.0147) (4.1053, 7.7471) knots 0 0 0 1 2 2 2
  line L352 (4.1053, 7.7471) -> (4.3265, 7.6956)
  line L353 (4.3265, 7.6956) -> (4.3265, 6.9443)
  line L354 (4.3265, 6.9443) -> (-2.3065, 6.9443)
  line L355 (-2.3065, 6.9443) -> (-2.3065, 7.7471)
  line L356 (-2.3065, 7.7471) -> (0.0606, 7.7471)
  spline S438 degree 2 poles (0.0606, 7.7471) (-0.2121, 8.0507) (-0.5723, 8.7557) (-0.5723, 9.2034) knots 0 0 0 1 2 2 2
  spline S439 degree 2 poles (-0.5723, 9.2034) (-0.5723, 10.0113) (0.7193, 10.9375) (1.8668, 10.9375) knots 0 0 0 1 2 2 2
  spline S440 degree 2 poles (1.9286, 10.1091) (1.0743, 10.1091) (0.1893, 9.5893) (0.1893, 9.013) knots 0 0 0 1 2 2 2
  spline S441 degree 2 poles (0.1893, 9.013) (0.1893, 8.6888) (0.498, 8.0198) (0.7347, 7.7471) knots 0 0 0 1 2 2 2
  line L357 (0.7347, 7.7471) -> (3.4672, 7.7471)
  spline S442 degree 2 poles (3.4672, 7.7471) (3.6164, 8.0507) (3.7399, 8.519) (3.7399, 8.7969) knots 0 0 0 1 2 2 2
  spline S443 degree 2 poles (3.7399, 8.7969) (3.7399, 9.4092) (2.8702, 10.1091) (1.9286, 10.1091) knots 0 0 0 1 2 2 2
  spline S444 degree 2 poles (4.4346, 13.8398) (4.4346, 12.6974) (3.1533, 11.4418) (1.9697, 11.4418) knots 0 0 0 1 2 2 2
  spline S445 degree 2 poles (1.9697, 11.4418) (0.8068, 11.4418) (-0.5723, 12.6614) (-0.5723, 13.6443) knots 0 0 0 1 2 2 2
  spline S446 degree 2 poles (-0.5723, 13.6443) (-0.5723, 14.0868) (-0.315, 14.7712) (-0.0423, 15.0234) knots 0 0 0 1 2 2 2
  spline S447 degree 2 poles (-0.0423, 15.0234) (0.2304, 15.2807) (1.0177, 15.5534) (1.5889, 15.5534) knots 0 0 0 1 2 2 2
  line L358 (1.5889, 15.5534) -> (2.0263, 15.5534)
  line L359 (2.0263, 15.5534) -> (2.0263, 12.2549)
  spline S448 degree 2 poles (2.0263, 12.2549) (2.8548, 12.2549) (3.7348, 13.0885) (3.7348, 13.8295) knots 0 0 0 1 2 2 2
  spline S449 degree 2 poles (3.7348, 13.8295) (3.7348, 14.092) (3.6164, 14.6014) (3.5238, 14.8072) knots 0 0 0 1 2 2 2
  spline S450 degree 2 poles (3.5238, 14.8072) (3.4209, 15.0234) (3.2408, 15.3218) (3.1584, 15.4196) knots 0 0 0 1 2 2 2
  line L360 (3.1584, 15.4196) -> (3.1584, 15.4659)
  line L361 (3.1584, 15.4659) -> (4.0332, 15.4659)
  spline S451 degree 2 poles (4.0332, 15.4659) (4.0898, 15.327) (4.2545, 14.905) (4.3008, 14.7403) knots 0 0 0 1 2 2 2
  spline S452 degree 2 poles (4.3008, 14.7403) (4.3677, 14.5088) (4.4346, 14.128) (4.4346, 13.8398) knots 0 0 0 1 2 2 2
  spline S453 degree 2 poles (1.414, 14.7712) (1.0898, 14.7609) (0.6164, 14.6271) (0.4568, 14.4985) knots 0 0 0 1 2 2 2
  spline S454 degree 2 poles (0.4568, 14.4985) (0.2767, 14.3595) (0.0863, 13.9221) (0.0863, 13.598) knots 0 0 0 1 2 2 2
  spline S455 degree 2 poles (0.0863, 13.598) (0.0863, 13.2789) (0.2767, 12.8312) (0.462, 12.646) knots 0 0 0 1 2 2 2
  spline S456 degree 2 poles (0.462, 12.646) (0.6524, 12.4659) (1.1104, 12.2806) (1.414, 12.2549) knots 0 0 0 1 2 2 2
  line L362 (1.414, 12.2549) -> (1.414, 14.7712)
  spline S457 degree 2 poles (2.3762, 20.7353) (2.8497, 20.7353) (3.5752, 20.3751) (3.8119, 20.0766) knots 0 0 0 1 2 2 2
  spline S458 degree 2 poles (3.8119, 20.0766) (4.0898, 19.7164) (4.3265, 18.8982) (4.3265, 18.2498) knots 0 0 0 1 2 2 2
  line L363 (4.3265, 18.2498) -> (4.3265, 16.4282)
  line L364 (4.3265, 16.4282) -> (-2.0235, 16.4282)
  line L365 (-2.0235, 16.4282) -> (-2.0235, 18.1109)
  spline S459 degree 2 poles (-2.0235, 18.1109) (-2.0235, 18.7901) (-1.936, 19.4694) (-1.7662, 19.7781) knots 0 0 0 1 2 2 2
  spline S460 degree 2 poles (-1.7662, 19.7781) (-1.5861, 20.1229) (-0.9943, 20.4368) (-0.5929, 20.4368) knots 0 0 0 1 2 2 2
  spline S461 degree 2 poles (-0.5929, 20.4368) (-0.1452, 20.4368) (0.5649, 19.9634) (0.7656, 19.5466) knots 0 0 0 1 2 2 2
  line L366 (0.7656, 19.5466) -> (0.7965, 19.5466)
  spline S462 degree 2 poles (0.7965, 19.5466) (0.9508, 20.1126) (1.769, 20.7353) (2.3762, 20.7353) knots 0 0 0 1 2 2 2
  spline S463 degree 2 poles (2.4123, 19.8553) (2.0521, 19.8553) (1.5889, 19.6495) (1.4243, 19.3407) knots 0 0 0 1 2 2 2
  spline S464 degree 2 poles (1.4243, 19.3407) (1.3213, 19.1401) (1.2596, 18.6666) (1.2596, 18.2292) knots 0 0 0 1 2 2 2
  line L367 (1.2596, 18.2292) -> (1.2596, 17.2721)
  line L368 (1.2596, 17.2721) -> (3.6061, 17.2721)
  line L369 (3.6061, 17.2721) -> (3.6061, 17.9565)
  spline S465 degree 2 poles (3.6061, 17.9565) (3.6061, 18.5123) (3.5032, 19.1503) (3.3385, 19.3973) knots 0 0 0 1 2 2 2
  spline S466 degree 2 poles (3.3385, 19.3973) (3.1687, 19.6341) (2.7467, 19.8553) (2.4123, 19.8553) knots 0 0 0 1 2 2 2
  spline S467 degree 2 poles (-0.4746, 19.5569) (-0.701, 19.5569) (-1.0406, 19.4025) (-1.1384, 19.2327) knots 0 0 0 1 2 2 2
  spline S468 degree 2 poles (-1.1384, 19.2327) (-1.2516, 19.0268) (-1.3031, 18.5277) (-1.3031, 18.08) knots 0 0 0 1 2 2 2
  line L370 (-1.3031, 18.08) -> (-1.3031, 17.2721)
  line L371 (-1.3031, 17.2721) -> (0.5546, 17.2721)
  line L372 (0.5546, 17.2721) -> (0.5546, 18.2292)
  spline S469 degree 2 poles (0.5546, 18.2292) (0.5546, 18.6255) (0.4723, 19.0011) (0.3436, 19.2018) knots 0 0 0 1 2 2 2
  spline S470 degree 2 poles (0.3436, 19.2018) (0.2201, 19.3973) (-0.1761, 19.5569) (-0.4746, 19.5569) knots 0 0 0 1 2 2 2
  line L373 (0.4208, 24.0389) -> (0.4208, 23.9978)
  spline S471 degree 2 poles (0.4208, 23.9978) (0.3951, 23.9051) (0.3848, 23.7044) (0.3848, 23.5655) knots 0 0 0 1 2 2 2
  spline S472 degree 2 poles (0.3848, 23.5655) (0.3848, 23.2413) (0.6678, 22.6032) (0.9457, 22.3151) knots 0 0 0 1 2 2 2
  line L374 (0.9457, 22.3151) -> (4.3265, 22.3151)
  line L375 (4.3265, 22.3151) -> (4.3265, 21.5123)
  line L376 (4.3265, 21.5123) -> (-0.4385, 21.5123)
  line L377 (-0.4385, 21.5123) -> (-0.4385, 22.3151)
  line L378 (-0.4385, 22.3151) -> (0.2716, 22.3151)
  spline S473 degree 2 poles (0.2716, 22.3151) (-0.1195, 22.7525) (-0.4385, 23.406) (-0.4385, 23.7147) knots 0 0 0 1 2 2 2
  spline S474 degree 2 poles (-0.4385, 23.7147) (-0.4385, 23.8382) (-0.4283, 23.9617) (-0.4128, 24.0389) knots 0 0 0 1 2 2 2
  line L379 (-0.4128, 24.0389) -> (0.4208, 24.0389)
  spline S475 degree 2 poles (3.8222, 27.3168) (3.8943, 27.2191) (4.1516, 26.8897) (4.2288, 26.7354) knots 0 0 0 1 2 2 2
  spline S476 degree 2 poles (4.2288, 26.7354) (4.342, 26.5244) (4.4603, 26.1281) (4.4603, 25.7679) knots 0 0 0 1 2 2 2
  spline S477 degree 2 poles (4.4603, 25.7679) (4.4603, 25.4746) (4.239, 24.9446) (4.0384, 24.7439) knots 0 0 0 1 2 2 2
  spline S478 degree 2 poles (4.0384, 24.7439) (3.8428, 24.5535) (3.2665, 24.3219) (2.9474, 24.3219) knots 0 0 0 1 2 2 2
  spline S479 degree 2 poles (2.9474, 24.3219) (2.4534, 24.3219) (1.7536, 24.7388) (1.5529, 25.1916) knots 0 0 0 1 2 2 2
  spline S480 degree 2 poles (1.5529, 25.1916) (1.3677, 25.593) (1.2287, 26.6839) (1.1927, 27.3168) knots 0 0 0 1 2 2 2
  line L380 (1.1927, 27.3168) -> (1.0383, 27.3168)
  spline S481 degree 2 poles (1.0383, 27.3168) (0.7604, 27.3168) (0.4157, 27.147) (0.3179, 26.9926) knots 0 0 0 1 2 2 2
  spline S482 degree 2 poles (0.3179, 26.9926) (0.2201, 26.8383) (0.1584, 26.3957) (0.1584, 26.159) knots 0 0 0 1 2 2 2
  spline S483 degree 2 poles (0.1584, 26.159) (0.1584, 25.8811) (0.323, 25.1298) (0.4826, 24.7542) knots 0 0 0 1 2 2 2
  line L381 (0.4826, 24.7542) -> (0.4826, 24.7079)
  line L382 (0.4826, 24.7079) -> (-0.3356, 24.7079)
  spline S484 degree 2 poles (-0.3356, 24.7079) (-0.3974, 24.9292) (-0.5518, 25.7576) (-0.5518, 26.1642) knots 0 0 0 1 2 2 2
  spline S485 degree 2 poles (-0.5518, 26.1642) (-0.5518, 26.6582) (-0.3974, 27.3323) (-0.1967, 27.5999) knots 0 0 0 1 2 2 2
  spline S486 degree 2 poles (-0.1967, 27.5999) (-0.0011, 27.8623) (0.6215, 28.1196) (1.0692, 28.1196) knots 0 0 0 1 2 2 2
  line L383 (1.0692, 28.1196) -> (4.3265, 28.1196)
  line L384 (4.3265, 28.1196) -> (4.3265, 27.3168)
  line L385 (4.3265, 27.3168) -> (3.8222, 27.3168)
  line L386 (3.1533, 27.3168) -> (1.8308, 27.3168)
  spline S487 degree 2 poles (1.8308, 27.3168) (1.8565, 27.0287) (1.944, 26.159) (2.0263, 25.8863) knots 0 0 0 1 2 2 2
  spline S488 degree 2 poles (2.0263, 25.8863) (2.1241, 25.5672) (2.5306, 25.1504) (2.8908, 25.1504) knots 0 0 0 1 2 2 2
  spline S489 degree 2 poles (2.8908, 25.1504) (3.3025, 25.1504) (3.7193, 25.6136) (3.7193, 26.0561) knots 0 0 0 1 2 2 2
  spline S490 degree 2 poles (3.7193, 26.0561) (3.7193, 26.4317) (3.3951, 27.0493) (3.1533, 27.3168) knots 0 0 0 1 2 2 2
  spline S491 degree 2 poles (4.4346, 31.1402) (4.4346, 30.6462) (4.131, 29.828) (3.8222, 29.5347) knots 0 0 0 1 2 2 2
  spline S492 degree 2 poles (3.8222, 29.5347) (3.5186, 29.2414) (2.5821, 28.9172) (1.9543, 28.9172) knots 0 0 0 1 2 2 2
  spline S493 degree 2 poles (1.9543, 28.9172) (1.3265, 28.9172) (0.4105, 29.2517) (0.1018, 29.5347) knots 0 0 0 1 2 2 2
  spline S494 degree 2 poles (0.1018, 29.5347) (-0.2121, 29.8177) (-0.5466, 30.6565) (-0.5466, 31.1402) knots 0 0 0 1 2 2 2
  spline S495 degree 2 poles (-0.5466, 31.1402) (-0.5466, 31.5313) (-0.3253, 32.262) (-0.1813, 32.545) knots 0 0 0 1 2 2 2
  line L387 (-0.1813, 32.545) -> (0.7193, 32.545)
  line L388 (0.7193, 32.545) -> (0.7193, 32.4987)
  spline S496 degree 2 poles (0.7193, 32.4987) (0.6472, 32.4112) (0.462, 32.1437) (0.3642, 31.9533) knots 0 0 0 1 2 2 2
  spline S497 degree 2 poles (0.3642, 31.9533) (0.2819, 31.7834) (0.1532, 31.3306) (0.1532, 31.1248) knots 0 0 0 1 2 2 2
  spline S498 degree 2 poles (0.1532, 31.1248) (0.1532, 30.5021) (1.0949, 29.7457) (1.9543, 29.7457) knots 0 0 0 1 2 2 2
  spline S499 degree 2 poles (1.9543, 29.7457) (2.7931, 29.7457) (3.7348, 30.4764) (3.7348, 31.1248) knots 0 0 0 1 2 2 2
  spline S500 degree 2 poles (3.7348, 31.1248) (3.7348, 31.5159) (3.4106, 32.226) (3.1584, 32.4987) knots 0 0 0 1 2 2 2
  line L389 (3.1584, 32.4987) -> (3.1584, 32.545)
  line L390 (3.1584, 32.545) -> (4.0589, 32.545)
  spline S501 degree 2 poles (4.0589, 32.545) (4.1155, 32.4267) (4.2751, 32.0665) (4.3111, 31.9224) knots 0 0 0 1 2 2 2
  spline S502 degree 2 poles (4.3111, 31.9224) (4.3728, 31.7166) (4.4346, 31.3924) (4.4346, 31.1402) knots 0 0 0 1 2 2 2
  line L391 (4.3265, 37.2226) -> (4.3265, 36.1677)
  line L392 (4.3265, 36.1677) -> (2.0263, 34.3975)
  line L393 (2.0263, 34.3975) -> (2.3351, 34.0785)
  line L394 (2.3351, 34.0785) -> (4.3265, 34.0785)
  line L395 (4.3265, 34.0785) -> (4.3265, 33.2757)
  line L396 (4.3265, 33.2757) -> (-2.3065, 33.2757)
  line L397 (-2.3065, 33.2757) -> (-2.3065, 34.0785)
  line L398 (-2.3065, 34.0785) -> (1.5735, 34.0785)
  line L399 (1.5735, 34.0785) -> (-0.4385, 35.9619)
  line L400 (-0.4385, 35.9619) -> (-0.4385, 36.9602)
  line L401 (-0.4385, 36.9602) -> (1.5529, 35.0048)
  line L402 (1.5529, 35.0048) -> (4.3265, 37.2226)
  spline S503 degree 2 poles (4.4346, 39.6926) (4.4346, 38.5503) (3.1533, 37.2947) (1.9697, 37.2947) knots 0 0 0 1 2 2 2
  spline S504 degree 2 poles (1.9697, 37.2947) (0.8068, 37.2947) (-0.5723, 38.5142) (-0.5723, 39.4971) knots 0 0 0 1 2 2 2
  spline S505 degree 2 poles (-0.5723, 39.4971) (-0.5723, 39.9396) (-0.315, 40.624) (-0.0423, 40.8762) knots 0 0 0 1 2 2 2
  spline S506 degree 2 poles (-0.0423, 40.8762) (0.2304, 41.1335) (1.0177, 41.4062) (1.5889, 41.4062) knots 0 0 0 1 2 2 2
  line L403 (1.5889, 41.4062) -> (2.0263, 41.4062)
  line L404 (2.0263, 41.4062) -> (2.0263, 38.1077)
  spline S507 degree 2 poles (2.0263, 38.1077) (2.8548, 38.1077) (3.7348, 38.9413) (3.7348, 39.6824) knots 0 0 0 1 2 2 2
  spline S508 degree 2 poles (3.7348, 39.6824) (3.7348, 39.9448) (3.6164, 40.4542) (3.5238, 40.6601) knots 0 0 0 1 2 2 2
  spline S509 degree 2 poles (3.5238, 40.6601) (3.4209, 40.8762) (3.2408, 41.1747) (3.1584, 41.2724) knots 0 0 0 1 2 2 2
  line L405 (3.1584, 41.2724) -> (3.1584, 41.3187)
  line L406 (3.1584, 41.3187) -> (4.0332, 41.3187)
  spline S510 degree 2 poles (4.0332, 41.3187) (4.0898, 41.1798) (4.2545, 40.7578) (4.3008, 40.5932) knots 0 0 0 1 2 2 2
  spline S511 degree 2 poles (4.3008, 40.5932) (4.3677, 40.3616) (4.4346, 39.9808) (4.4346, 39.6926) knots 0 0 0 1 2 2 2
  spline S512 degree 2 poles (1.414, 40.624) (1.0898, 40.6138) (0.6164, 40.48) (0.4568, 40.3513) knots 0 0 0 1 2 2 2
  spline S513 degree 2 poles (0.4568, 40.3513) (0.2767, 40.2124) (0.0863, 39.775) (0.0863, 39.4508) knots 0 0 0 1 2 2 2
  spline S514 degree 2 poles (0.0863, 39.4508) (0.0863, 39.1317) (0.2767, 38.6841) (0.462, 38.4988) knots 0 0 0 1 2 2 2
  spline S515 degree 2 poles (0.462, 38.4988) (0.6524, 38.3187) (1.1104, 38.1334) (1.414, 38.1077) knots 0 0 0 1 2 2 2
  line L407 (1.414, 38.1077) -> (1.414, 40.624)
  spline S516 degree 2 poles (4.4192, 43.6601) (4.4192, 43.0066) (3.673, 42.2707) (2.8651, 42.2707) knots 0 0 0 1 2 2 2
  line L408 (2.8651, 42.2707) -> (0.2253, 42.2707)
  line L409 (0.2253, 42.2707) -> (0.2253, 41.7304)
  line L410 (0.2253, 41.7304) -> (-0.4385, 41.7304)
  line L411 (-0.4385, 41.7304) -> (-0.4385, 42.2707)
  line L412 (-0.4385, 42.2707) -> (-1.8073, 42.2707)
  line L413 (-1.8073, 42.2707) -> (-1.8073, 43.0735)
  line L414 (-1.8073, 43.0735) -> (-0.4385, 43.0735)
  line L415 (-0.4385, 43.0735) -> (-0.4385, 44.5503)
  line L416 (-0.4385, 44.5503) -> (0.2253, 44.5503)
  line L417 (0.2253, 44.5503) -> (0.2253, 43.0735)
  line L418 (0.2253, 43.0735) -> (2.4946, 43.0735)
  spline S517 degree 2 poles (2.4946, 43.0735) (2.8548, 43.0735) (3.251, 43.0992) (3.4209, 43.1867) knots 0 0 0 1 2 2 2
  spline S518 degree 2 poles (3.4209, 43.1867) (3.5701, 43.2587) (3.7193, 43.5829) (3.7193, 43.8608) knots 0 0 0 1 2 2 2
  spline S519 degree 2 poles (3.7193, 43.8608) (3.7193, 44.0563) (3.601, 44.4217) (3.5649, 44.504) knots 0 0 0 1 2 2 2
  line L419 (3.5649, 44.504) -> (3.5649, 44.5503)
  line L420 (3.5649, 44.5503) -> (4.2854, 44.5503)
  spline S520 degree 2 poles (4.2854, 44.5503) (4.3471, 44.3239) (4.4192, 43.8608) (4.4192, 43.6601) knots 0 0 0 1 2 2 2
  spline S521 degree 2 poles (4.4397, 47.6842) (4.4397, 47.0667) (4.0229, 46.0221) (3.6061, 45.6413) knots 0 0 0 1 2 2 2
  spline S522 degree 2 poles (3.6061, 45.6413) (3.1944, 45.2605) (1.9594, 44.8437) (1.1567, 44.8437) knots 0 0 0 1 2 2 2
  spline S523 degree 2 poles (1.1567, 44.8437) (0.3591, 44.8437) (-0.8245, 45.2502) (-1.2619, 45.6361) knots 0 0 0 1 2 2 2
  spline S524 degree 2 poles (-1.2619, 45.6361) (-1.689, 46.0169) (-2.1367, 47.0564) (-2.1367, 47.6996) knots 0 0 0 1 2 2 2
  spline S525 degree 2 poles (-2.1367, 47.6996) (-2.1367, 48.0187) (-2.0441, 48.5796) (-1.972, 48.8163) knots 0 0 0 1 2 2 2
  spline S526 degree 2 poles (-1.972, 48.8163) (-1.9051, 49.0221) (-1.7147, 49.4492) (-1.6015, 49.6602) knots 0 0 0 1 2 2 2
  line L421 (-1.6015, 49.6602) -> (-0.5826, 49.6602)
  line L422 (-0.5826, 49.6602) -> (-0.5826, 49.5933)
  spline S527 degree 2 poles (-0.5826, 49.5933) (-0.6855, 49.4801) (-0.9737, 49.1302) (-1.1127, 48.878) knots 0 0 0 1 2 2 2
  spline S528 degree 2 poles (-1.1127, 48.878) (-1.2464, 48.6362) (-1.4163, 48.065) (-1.4163, 47.6945) knots 0 0 0 1 2 2 2
  spline S529 degree 2 poles (-1.4163, 47.6945) (-1.4163, 47.2879) (-1.0818, 46.5624) (-0.7627, 46.2896) knots 0 0 0 1 2 2 2
  spline S530 degree 2 poles (-0.7627, 46.2896) (-0.4385, 46.0221) (0.5443, 45.7236) (1.1567, 45.7236) knots 0 0 0 1 2 2 2
  spline S531 degree 2 poles (1.1567, 45.7236) (1.8102, 45.7236) (2.7519, 46.0375) (3.0761, 46.3102) knots 0 0 0 1 2 2 2
  spline S532 degree 2 poles (3.0761, 46.3102) (3.39, 46.5778) (3.709, 47.2931) (3.709, 47.6945) knots 0 0 0 1 2 2 2
  spline S533 degree 2 poles (3.709, 47.6945) (3.709, 48.0598) (3.5289, 48.6825) (3.3951, 48.9243) knots 0 0 0 1 2 2 2
  spline S534 degree 2 poles (3.3951, 48.9243) (3.2613, 49.1559) (2.9835, 49.5007) (2.8857, 49.5984) knots 0 0 0 1 2 2 2
  line L423 (2.8857, 49.5984) -> (2.8857, 49.6602)
  line L424 (2.8857, 49.6602) -> (3.8943, 49.6602)
  spline S535 degree 2 poles (3.8943, 49.6602) (3.992, 49.4492) (4.1722, 49.0787) (4.2545, 48.8163) knots 0 0 0 1 2 2 2
  spline S536 degree 2 poles (4.2545, 48.8163) (4.3471, 48.5384) (4.4397, 48.065) (4.4397, 47.6842) knots 0 0 0 1 2 2 2
  line L425 (0.4208, 52.9124) -> (0.4208, 52.8712)
  spline S537 degree 2 poles (0.4208, 52.8712) (0.3951, 52.7786) (0.3848, 52.5779) (0.3848, 52.439) knots 0 0 0 1 2 2 2
  spline S538 degree 2 poles (0.3848, 52.439) (0.3848, 52.1148) (0.6678, 51.4767) (0.9457, 51.1885) knots 0 0 0 1 2 2 2
  line L426 (0.9457, 51.1885) -> (4.3265, 51.1885)
  line L427 (4.3265, 51.1885) -> (4.3265, 50.3858)
  line L428 (4.3265, 50.3858) -> (-0.4385, 50.3858)
  line L429 (-0.4385, 50.3858) -> (-0.4385, 51.1885)
  line L430 (-0.4385, 51.1885) -> (0.2716, 51.1885)
  spline S539 degree 2 poles (0.2716, 51.1885) (-0.1195, 51.6259) (-0.4385, 52.2794) (-0.4385, 52.5882) knots 0 0 0 1 2 2 2
  spline S540 degree 2 poles (-0.4385, 52.5882) (-0.4385, 52.7117) (-0.4283, 52.8352) (-0.4128, 52.9124) knots 0 0 0 1 2 2 2
  line L431 (-0.4128, 52.9124) -> (0.4208, 52.9124)
  spline S541 degree 2 poles (3.8222, 56.1903) (3.8943, 56.0925) (4.1516, 55.7632) (4.2288, 55.6088) knots 0 0 0 1 2 2 2
  spline S542 degree 2 poles (4.2288, 55.6088) (4.342, 55.3978) (4.4603, 55.0016) (4.4603, 54.6414) knots 0 0 0 1 2 2 2
  spline S543 degree 2 poles (4.4603, 54.6414) (4.4603, 54.3481) (4.239, 53.818) (4.0384, 53.6174) knots 0 0 0 1 2 2 2
  spline S544 degree 2 poles (4.0384, 53.6174) (3.8428, 53.427) (3.2665, 53.1954) (2.9474, 53.1954) knots 0 0 0 1 2 2 2
  spline S545 degree 2 poles (2.9474, 53.1954) (2.4534, 53.1954) (1.7536, 53.6122) (1.5529, 54.0651) knots 0 0 0 1 2 2 2
  spline S546 degree 2 poles (1.5529, 54.0651) (1.3677, 54.4664) (1.2287, 55.5574) (1.1927, 56.1903) knots 0 0 0 1 2 2 2
  line L432 (1.1927, 56.1903) -> (1.0383, 56.1903)
  spline S547 degree 2 poles (1.0383, 56.1903) (0.7604, 56.1903) (0.4157, 56.0205) (0.3179, 55.8661) knots 0 0 0 1 2 2 2
  spline S548 degree 2 poles (0.3179, 55.8661) (0.2201, 55.7117) (0.1584, 55.2692) (0.1584, 55.0325) knots 0 0 0 1 2 2 2
  spline S549 degree 2 poles (0.1584, 55.0325) (0.1584, 54.7546) (0.323, 54.0033) (0.4826, 53.6277) knots 0 0 0 1 2 2 2
  line L433 (0.4826, 53.6277) -> (0.4826, 53.5813)
  line L434 (0.4826, 53.5813) -> (-0.3356, 53.5813)
  spline S550 degree 2 poles (-0.3356, 53.5813) (-0.3974, 53.8026) (-0.5518, 54.6311) (-0.5518, 55.0376) knots 0 0 0 1 2 2 2
  spline S551 degree 2 poles (-0.5518, 55.0376) (-0.5518, 55.5316) (-0.3974, 56.2057) (-0.1967, 56.4733) knots 0 0 0 1 2 2 2
  spline S552 degree 2 poles (-0.1967, 56.4733) (-0.0011, 56.7358) (0.6215, 56.993) (1.0692, 56.993) knots 0 0 0 1 2 2 2
  line L435 (1.0692, 56.993) -> (4.3265, 56.993)
  line L436 (4.3265, 56.993) -> (4.3265, 56.1903)
  line L437 (4.3265, 56.1903) -> (3.8222, 56.1903)
  line L438 (3.1533, 56.1903) -> (1.8308, 56.1903)
  spline S553 degree 2 poles (1.8308, 56.1903) (1.8565, 55.9021) (1.944, 55.0325) (2.0263, 54.7597) knots 0 0 0 1 2 2 2
  spline S554 degree 2 poles (2.0263, 54.7597) (2.1241, 54.4407) (2.5306, 54.0239) (2.8908, 54.0239) knots 0 0 0 1 2 2 2
  spline S555 degree 2 poles (2.8908, 54.0239) (3.3025, 54.0239) (3.7193, 54.487) (3.7193, 54.9296) knots 0 0 0 1 2 2 2
  spline S556 degree 2 poles (3.7193, 54.9296) (3.7193, 55.3052) (3.3951, 55.9227) (3.1533, 56.1903) knots 0 0 0 1 2 2 2
  line L439 (4.3265, 61.7839) -> (4.3265, 60.9811)
  line L440 (4.3265, 60.9811) -> (3.8428, 60.9811)
  spline S557 degree 2 poles (3.8428, 60.9811) (3.9972, 60.7958) (4.203, 60.5231) (4.2905, 60.3379) knots 0 0 0 1 2 2 2
  spline S558 degree 2 poles (4.2905, 60.3379) (4.3728, 60.168) (4.4603, 59.8027) (4.4603, 59.5608) knots 0 0 0 1 2 2 2
  spline S559 degree 2 poles (4.4603, 59.5608) (4.4603, 59.1698) (4.1361, 58.5111) (3.8222, 58.2795) knots 0 0 0 1 2 2 2
  spline S560 degree 2 poles (3.8222, 58.2795) (3.5083, 58.048) (2.5821, 57.7907) (1.98, 57.7907) knots 0 0 0 1 2 2 2
  spline S561 degree 2 poles (1.98, 57.7907) (1.3522, 57.7907) (0.4363, 58.1148) (0.0915, 58.3979) knots 0 0 0 1 2 2 2
  spline S562 degree 2 poles (0.0915, 58.3979) (-0.2173, 58.6603) (-0.5723, 59.3962) (-0.5723, 59.8027) knots 0 0 0 1 2 2 2
  spline S563 degree 2 poles (-0.5723, 59.8027) (-0.5723, 60.1578) (-0.4128, 60.6878) (-0.2481, 60.9811) knots 0 0 0 1 2 2 2
  line L441 (-0.2481, 60.9811) -> (-2.3065, 60.9811)
  line L442 (-2.3065, 60.9811) -> (-2.3065, 61.7839)
  line L443 (-2.3065, 61.7839) -> (4.3265, 61.7839)
  line L444 (3.1687, 60.9811) -> (0.4157, 60.9811)